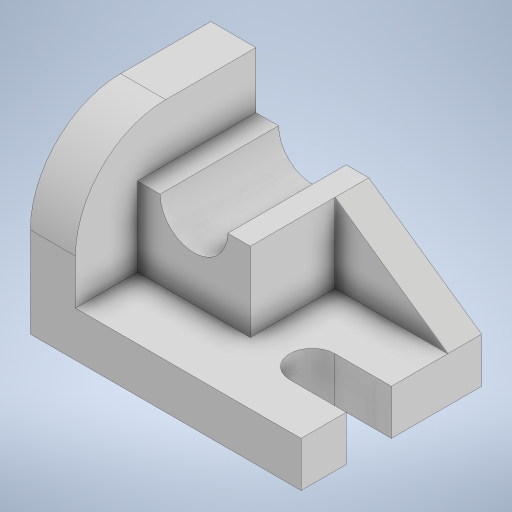
# Autodesk Inventor part: 1
Saved by Autodesk Inventor 2023 (Build 270158000, 158)
## iProperties
Created: 2023-09-26
Part Number: 1
Material: Všeobecné
Document SubType Name: Modeling
Designer: clu40164
Mass: 181.471 g
Surface Area: 276.267 cm^2
Volume: 181.471 cm^3
Density: 1 g/cm^3
Appearance: Výchozí
Author: clu40164
Autodesk Inventor part; units mm, degrees
ref_plane "YZ Plane" through (0, 0, 0) normal (1, 0, 0) x (0, 1, 0)
ref_plane "XZ Plane" through (0, 0, 0) normal (0, 1, 0) x (-1, 0, 0)
ref_plane "XY Plane" through (0, 0, 0) normal (0, 0, 1) x (1, 0, 0)
sketch "Náčrt1" plane through (0, 0, 0) normal (0, 1, 0) x (-1, 0, 0)
  line L0 (48, 32) -> (-48, 32)
  line L1 (-48, -32) -> (48, -32)
  line L2 (48, -32) -> (48, 32)
  line L3 (48, 32) -> (-48, -32) construction
  line L4 (-48, 32) -> (48, -32) construction
  line L5 (-48, 32) -> (-48, 16)
  line L6 (-48, 16) -> (-28, 16)
  line L7 (-48, 0) -> (-48, -32)
  line L8 (-48, 0) -> (-28, 0)
  arc A0 (-28, 0) -> (-28, 16) centre (-28, 8) ccw
  point P0 (0, 0)
  dimension "d0" = 96
  dimension "d1" = 16
  dimension "d2" = 20
  dimension "d3" = 16
  dimension "d4" = 8
  dimension "d5" = 64
  dimension "d6" = 8
  dimension "d9" = 76
  dimension "d10" = 76
  constraints: 18 end point, 2 horizontal, 2 midpoint, 2 point on circle, 2 vertical, 1 centre point, 1 collinear, 1 parallel, 1 perpendicular
  measures "d0" distance of L0.start L0.end
  measures "d1" distance of L0.end L5.end
  measures "d2" distance of L5.end L6.end
  measures "d3" distance of L7.start L5.end
  measures "d4" distance of A0.centre L6.end
  measures "d5" distance of L1.end L0.start
  measures "d6" distance of L8.end A0.centre
  measures "d9" distance from line of A0.centre L2
  measures "d10" distance from line of A0.start L2
extrude "Vysunutí1" add sketch "Náčrt1" along normal blind 16
sketch "Náčrt3" plane through (-48, 0, -32) normal (-1, 0, 0) x (0, 0, 1)
  line L0 (32, 16) -> (0, 16) projected
  line L1 (0, 16) -> (64, 16)
  line L2 (64, 16) -> (64, 32)
  line L3 (32, 64) -> (0, 64)
  line L4 (0, 64) -> (0, 16)
  arc A0 (64, 32) -> (32, 64) centre (32, 32) ccw
  point P0 (32, 0)
  point P1 (64, 64)
  dimension "d13" = 48
  dimension "d14" = 64
  dimension "d15" = 32
  constraints: 8 end point, 2 parallel, 2 point on circle, 2 point on line, 2 tangent, 1 centre point, 1 horizontal, 1 perpendicular
  measures "d13" distance of L1.end point (64, 64)
  measures "d14" distance between parallel lines of L4 L2
  measures "d15" radius of A0
extrude "Vysunutí2" add sketch "Náčrt3" against normal blind 16
sketch "Náčrt4" plane through (48, 0, -32) normal (0, 0, -1) x (-1, 0, 0)
  line L0 (0, 16) -> (80, 16) projected
  line L1 (80, 16) -> (40, 16)
  line L2 (40, 16) -> (40, 44)
  line L3 (80, 44) -> (80, 16)
  line L4 (40, 44) -> (48, 44)
  line L5 (80, 44) -> (72, 44)
  arc A0 (48, 44) -> (72, 44) centre (60, 44) ccw
  point P0 (48, 0)
  dimension "d18" = 28
  dimension "d19" = 40
  dimension "d20" = 8
  dimension "d21" = 12
  dimension "d22" = 12
  dimension "d23" = 8
  dimension "d24" = 28
  constraints: 10 end point, 3 horizontal, 2 point on circle, 1 centre point, 1 parallel, 1 perpendicular, 1 point on line
  measures "d18" distance of L1.end L2.end
  measures "d19" distance of L2.end L3.start
  measures "d20" distance of L2.end L4.end
  measures "d21" distance of A0.centre L4.end
  measures "d22" distance of L5.end A0.centre
  measures "d23" distance of L3.start L5.end
  measures "d24" distance between parallel lines of L5 L0
extrude "Vysunutí3" add sketch "Náčrt4" against normal blind 42
sketch "Náčrt5" plane through (48, 0, -32) normal (0, 0, -1) x (-1, 0, 0)
  line L0 (40, 44) -> (0, 16)
  line L1 (0, 16) -> (40, 16)
  line L2 (40, 16) -> (40, 44)
  point P0 (48, 0)
  constraints: 6 end point, 3 coincident
extrude "Vysunutí4" add sketch "Náčrt5" against normal blind 12
